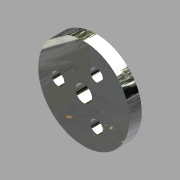
# Autodesk Inventor part: WheelAdapter-4mm-2
Saved by Autodesk Inventor 2017 (Build 210142000, 142)
## iProperties
Created: 2017-05-07
Part Number: WheelAdapter-4mm-2
Material: Aluminum 6061
Document SubType Name: Modeling
Designer: zallen
Density: 2.7 g/cm^3
Appearance: Aluminum - Flat
Mass: 2.80552 g
Surface Area: 10.2259 cm^2
Volume: 1.03908 cm^3
Author: zallen
Autodesk Inventor part; units mm, degrees
ref_plane "YZ Plane" through (0, 0, 0) normal (1, 0, 0) x (0, 1, 0)
ref_plane "XZ Plane" through (0, 0, 0) normal (0, 1, 0) x (-1, 0, 0)
ref_plane "XY Plane" through (0, 0, 0) normal (0, 0, 1) x (1, 0, 0)
sketch "Sketch1" plane through (0, 0, 0) normal (0, 0, 1) x (1, 0, 0)
  point P0 (0, 0)
sketch "Sketch2" plane through (0, 0, 0) normal (0, 0, 1) x (1, 0, 0)
  circle A0 centre (0, 0) radius 11
  circle A1 centre (0, 0) radius 2
  circle A2 centre (-6.2, 0) radius 1.5
  circle A3 centre (0, 0) radius 6.2 construction
  circle A4 centre (3.1, -5.3694) radius 1.5
  circle A5 centre (3.1, 5.3694) radius 1.5
  dimension "d3" = 12.4
  dimension "d0" = 22
  dimension "d1" = 4
  dimension "d2" = 3
  dimension "d6" = 360
  constraints: 5 centre point, 3 coincident, 1 horizontal alignment, 9 other
  measures "d0" diameter of A0
  measures "d1" diameter of A1
  measures "d2" diameter of A2
extrude "Extrusion1" add sketch "Sketch2" along normal blind 3
body "Solid1"
